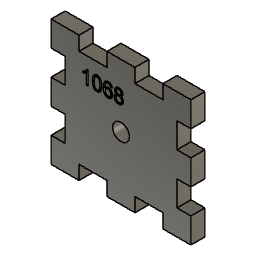
FullSystemAssembly (Autodesk Fusion 360 archive; units mm, degrees)
design "Housing_4"
Autodesk Fusion 360 part; units mm, degrees
(part 1 of 2)
sketch "Sketch1" plane through (0, 0, 0) normal (0, 1, 0) x (1, 0, 0)
  line L0 (-40.266, -48.8623) -> (-30.266, -48.8623)
  line L1 (-30.266, -48.8623) -> (-30.266, -43.8623)
  line L2 (-35.266, -39.8623) -> (-40.266, -39.8623)
  line L3 (-40.266, -39.8623) -> (-40.266, -48.8623)
  line L4 (-20.266, -48.8623) -> (-10.266, -48.8623)
  line L5 (-10.266, -48.8623) -> (-10.266, -43.8623)
  line L6 (-20.266, -43.8623) -> (-20.266, -48.8623)
  line L7 (-40.266, -30.8623) -> (-35.266, -30.8623)
  line L8 (-35.266, -21.8623) -> (-40.266, -21.8623)
  line L9 (-40.266, -21.8623) -> (-40.266, -30.8623)
  line L10 (-15.266, -66.877) -> (-15.266, -0.0799) construction
  line L11 (24.5212, -26.3623) -> (-48.7253, -26.3623) construction
  line L12 (4.734, -39.8623) -> (9.734, -39.8623)
  line L13 (-0.266, -48.8623) -> (-0.266, -43.8623)
  line L14 (9.734, -30.8623) -> (4.734, -30.8623)
  line L15 (4.734, -21.8623) -> (9.734, -21.8623)
  line L16 (-35.266, -12.8623) -> (-40.266, -12.8623)
  line L17 (-30.266, -3.8623) -> (-30.266, -8.8623)
  line L18 (-20.266, -8.8623) -> (-20.266, -3.8623)
  line L19 (-10.266, -3.8623) -> (-10.266, -8.8623)
  line L20 (-0.266, -3.8623) -> (-0.266, -8.8623)
  line L21 (4.734, -12.8623) -> (9.734, -12.8623)
  line L22 (-40.266, -48.8623) -> (-30.266, -48.8623)
  line L23 (-20.266, -48.8623) -> (-10.266, -48.8623)
  line L24 (-0.266, -48.8623) -> (9.734, -48.8623)
  line L25 (9.734, -48.8623) -> (9.734, -39.8623)
  line L26 (9.734, -30.8623) -> (9.734, -21.8623)
  line L27 (9.734, -12.8623) -> (9.734, -3.8623)
  line L28 (-40.266, -3.8623) -> (-40.266, -12.8623)
  line L29 (-40.266, -21.8623) -> (-40.266, -30.8623)
  line L30 (-40.266, -39.8623) -> (-40.266, -48.8623)
  line L31 (-35.266, -39.8623) -> (-35.266, -30.8623)
  line L32 (-35.266, -21.8623) -> (-35.266, -12.8623)
  line L33 (4.734, -39.8623) -> (4.734, -30.8623)
  line L34 (4.734, -21.8623) -> (4.734, -12.8623)
  line L35 (9.734, -3.8623) -> (-0.266, -3.8623)
  line L36 (-10.266, -3.8623) -> (-20.266, -3.8623)
  line L37 (-30.266, -3.8623) -> (-40.266, -3.8623)
  line L38 (-30.266, -8.8623) -> (-20.266, -8.8623)
  line L39 (-10.266, -8.8623) -> (-0.266, -8.8623)
  line L40 (-30.266, -43.8623) -> (-20.266, -43.8623)
  line L41 (-10.266, -43.8623) -> (-0.266, -43.8623)
  dimension "d1" = 50
  dimension "d2" = 45
  dimension "d3" = 10
  dimension "d4" = 9
  dimension "d5" = 10
  dimension "d6" = 10
  dimension "d7" = 5
  dimension "d8" = 9
  dimension "d9" = 5
  dimension "d10" = 9
  constraint horizontal L22
  constraint vertical L25
  constraint horizontal L35
  constraint vertical L28
  constraint horizontal L0
  constraint vertical L1
  constraint horizontal L2
  constraint vertical L3
  constraint horizontal L4
  constraint vertical L5
  constraint vertical L6
  constraint horizontal L7
  constraint horizontal L8
  constraint vertical L9
  constraint perpendicular L10 L35
  constraint perpendicular L11 L28
  constraint symmetric L0.end L10 L13.start
  constraint symmetric L2.end L10 L12.end
  constraint symmetric L7.start L10 L14.start
  constraint symmetric L7.end L10 L14.end
  constraint symmetric L8.start L10 L15.start
  constraint symmetric L8.end L10 L15.end
  constraint symmetric L0.end L11 L17.start
  constraint symmetric L2.end L11 L16.end
  constraint symmetric L4.start L11 L18.end
  constraint symmetric L4.end L11 L19.start
  constraint symmetric L5.end L11 L19.end
  constraint symmetric L6.start L11 L18.start
  constraint symmetric L11 L12.end L21.end
  constraint symmetric L11 L13.start L20.start
  constraint perpendicular L16 L31
  constraint perpendicular L21 L33
  constraint perpendicular L20 L38
  constraint perpendicular L13 L40
  constraint collinear L22 L23
  constraint collinear L23 L24
  constraint collinear L25 L26
  constraint collinear L26 L27
  constraint collinear L28 L29
  constraint collinear L29 L30
  constraint collinear L31 L32
  constraint collinear L33 L34
  constraint collinear L35 L36
  constraint collinear L36 L37
  constraint collinear L38 L39
  constraint collinear L40 L41
  measures "d1" distance of L0.start L24.end
  measures "d2" distance of L0.start L28.start
  measures "d3" distance of L0.start L0.end
  measures "d4" distance of L0.start L2.end
  measures "d5" distance of L0.end L4.start
  measures "d6" distance of L4.start L4.end
  measures "d7" distance of L4.start L6.start
  measures "d8" distance of L2.end L7.start
  measures "d9" distance of L7.start L7.end
  measures "d10" distance of L7.start L8.end
extrude "Extrude1" add sketch "Sketch1" along normal blind 5
sketch "Sketch2" plane through (0, 0, 0) normal (0, -1, 0) x (1, 0, 0)
  line L0 (-40.266, 39.8623) -> (-35.266, 39.8623)
  line L1 (-35.266, 39.8623) -> (-35.266, 30.8623)
  line L2 (-35.266, 30.8623) -> (-40.266, 30.8623)
  line L3 (-40.266, 30.8623) -> (-40.266, 21.8623)
  line L4 (-40.266, 21.8623) -> (-35.266, 21.8623)
  line L5 (-35.266, 21.8623) -> (-35.266, 12.8623)
  line L6 (-35.266, 12.8623) -> (-40.266, 12.8623)
  line L7 (-40.266, 12.8623) -> (-40.266, 3.8623)
  line L8 (-40.266, 3.8623) -> (-30.266, 3.8623)
  line L9 (-30.266, 3.8623) -> (-30.266, 8.8623)
  line L10 (-30.266, 8.8623) -> (-20.266, 8.8623)
  line L11 (-20.266, 8.8623) -> (-20.266, 3.8623)
  line L12 (-20.266, 3.8623) -> (-10.266, 3.8623)
  line L13 (-10.266, 3.8623) -> (-10.266, 8.8623)
  line L14 (-10.266, 8.8623) -> (-0.266, 8.8623)
  line L15 (-0.266, 8.8623) -> (-0.266, 3.8623)
  line L16 (-0.266, 3.8623) -> (9.734, 3.8623)
  line L17 (9.734, 3.8623) -> (9.734, 12.8623)
  line L18 (9.734, 12.8623) -> (4.734, 12.8623)
  line L19 (4.734, 12.8623) -> (4.734, 21.8623)
  line L20 (4.734, 21.8623) -> (9.734, 21.8623)
  line L21 (9.734, 21.8623) -> (9.734, 30.8623)
  line L22 (9.734, 30.8623) -> (4.734, 30.8623)
  line L23 (4.734, 30.8623) -> (4.734, 39.8623)
  line L24 (4.734, 39.8623) -> (9.734, 39.8623)
  line L25 (9.734, 39.8623) -> (9.734, 48.8623)
  line L26 (9.734, 48.8623) -> (-0.266, 48.8623)
  line L27 (-0.266, 48.8623) -> (-0.266, 43.8623)
  line L28 (-0.266, 43.8623) -> (-10.266, 43.8623)
  line L29 (-10.266, 43.8623) -> (-10.266, 48.8623)
  line L30 (-10.266, 48.8623) -> (-20.266, 48.8623)
  line L31 (-20.266, 48.8623) -> (-20.266, 43.8623)
  line L32 (-20.266, 43.8623) -> (-30.266, 43.8623)
  line L33 (-30.266, 43.8623) -> (-30.266, 48.8623)
  line L34 (-30.266, 48.8623) -> (-40.266, 48.8623)
  line L35 (-40.266, 48.8623) -> (-40.266, 39.8623)
  circle A0 centre (-15.266, 26.3623) radius 3
  dimension "d13" = 6
  dimension "d14" = 22.5
  dimension "d15" = 25
  measures "d13" diameter of A0
  measures "d14" distance of L12 A0.centre
  measures "d15" distance of L3 A0.centre
extrude "Extrude2" cut sketch "Sketch2" against normal blind 5 contours A0
sketch "Sketch3" plane through (0, 0, 0) normal (0, -1, 0) x (1, 0, 0)
  circle A0 centre (-15.266, 26.3623) radius 3
  line L0 (-40.266, 39.8623) -> (-35.266, 39.8623)
  line L1 (-35.266, 39.8623) -> (-35.266, 30.8623)
  line L2 (-35.266, 30.8623) -> (-40.266, 30.8623)
  line L3 (-40.266, 30.8623) -> (-40.266, 21.8623)
  line L4 (-40.266, 21.8623) -> (-35.266, 21.8623)
  line L5 (-35.266, 21.8623) -> (-35.266, 12.8623)
  line L6 (-35.266, 12.8623) -> (-40.266, 12.8623)
  line L7 (-40.266, 12.8623) -> (-40.266, 3.8623)
  line L8 (-40.266, 3.8623) -> (-30.266, 3.8623)
  line L9 (-30.266, 3.8623) -> (-30.266, 8.8623)
  line L10 (-30.266, 8.8623) -> (-20.266, 8.8623)
  line L11 (-20.266, 8.8623) -> (-20.266, 3.8623)
  line L12 (-20.266, 3.8623) -> (-10.266, 3.8623)
  line L13 (-10.266, 3.8623) -> (-10.266, 8.8623)
  line L14 (-10.266, 8.8623) -> (-0.266, 8.8623)
  line L15 (-0.266, 8.8623) -> (-0.266, 3.8623)
  line L16 (-0.266, 3.8623) -> (9.734, 3.8623)
  line L17 (9.734, 3.8623) -> (9.734, 12.8623)
  line L18 (9.734, 12.8623) -> (4.734, 12.8623)
  line L19 (4.734, 12.8623) -> (4.734, 21.8623)
  line L20 (4.734, 21.8623) -> (9.734, 21.8623)
  line L21 (9.734, 21.8623) -> (9.734, 30.8623)
  line L22 (9.734, 30.8623) -> (4.734, 30.8623)
  line L23 (4.734, 30.8623) -> (4.734, 39.8623)
  line L24 (4.734, 39.8623) -> (9.734, 39.8623)
  line L25 (9.734, 39.8623) -> (9.734, 48.8623)
  line L26 (9.734, 48.8623) -> (-0.266, 48.8623)
  line L27 (-0.266, 48.8623) -> (-0.266, 43.8623)
  line L28 (-0.266, 43.8623) -> (-10.266, 43.8623)
  line L29 (-10.266, 43.8623) -> (-10.266, 48.8623)
  line L30 (-10.266, 48.8623) -> (-20.266, 48.8623)
  line L31 (-20.266, 48.8623) -> (-20.266, 43.8623)
  line L32 (-20.266, 43.8623) -> (-30.266, 43.8623)
  line L33 (-30.266, 43.8623) -> (-30.266, 48.8623)
  line L34 (-30.266, 48.8623) -> (-40.266, 48.8623)
  line L35 (-40.266, 48.8623) -> (-40.266, 39.8623)
  line L36 (-28.8758, 34.3033) -> (-13.6356, 34.3033) construction
  line L37 (-13.6356, 34.3033) -> (-13.6356, 39.6747) construction
  line L38 (-13.6356, 39.6747) -> (-28.8758, 39.6747) construction
  line L39 (-28.8758, 39.6747) -> (-28.8758, 34.3033) construction
  dimension "d18" = 5
  text T0 "1068" font "Arial" height 5 align left top in box 15.2402 x 5.3713 at (-28.8758, 34.3033) x (1, 0) y (0, 1) spacing 1 kerned
emboss "Emboss1" depth -0.7 profiles "Sketch3" section 1 text T0 onto face at (-2.7731, 0, 18.4656)

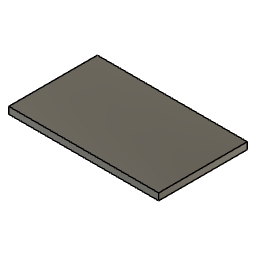
design "Base Plate"
Autodesk Fusion 360 part; units mm, degrees
sketch "Sketch1" plane through (0, 0, 0) normal (0, 0, 1) x (1, 0, 0)
  line L0 (-61.3423, 35.855) -> (48.6577, 35.855)
  line L1 (48.6577, 35.855) -> (48.6577, -29.145)
  line L2 (48.6577, -29.145) -> (-61.3423, -29.145)
  line L3 (-61.3423, -29.145) -> (-61.3423, 35.855)
  dimension "d1" = 110
  dimension "d2" = 65
  constraint horizontal L0
  constraint vertical L1
  constraint horizontal L2
  constraint vertical L3
  measures "d1" distance of L0.start L0.end
  measures "d2" distance of L0.start L2.end
extrude "Extrude1" add sketch "Sketch1" along normal blind 5

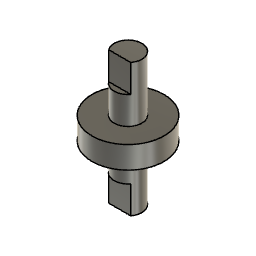
design "Shaft_bearing"
Autodesk Fusion 360 part; units mm, degrees
sketch "Sketch1" plane through (0, 0, 0) normal (0, 0, 1) x (1, 0, 0)
  circle A0 centre (0, 0) radius 6.5
  dimension "d1" = 13
  constraint coincident A0.centre origin
  measures "d1" diameter of A0
extrude "Extrude1" add sketch "Sketch1" along normal blind 4
sketch "Sketch2" plane through (0, 0, 4) normal (0, 0, 1) x (-1, 0, 0)
  circle A0 centre (0, 0) radius 6.5
  circle A1 centre (0, 0) radius 2.5
  dimension "d4" = 5
  constraint coincident A0.centre A1.centre
  measures "d4" diameter of A1
extrude "Extrude2" add sketch "Sketch2" along normal blind 5 contours A1
sketch "Sketch3" plane through (0, 0, 9) normal (0, 0, 1) x (-1, 0, 0)
  circle A0 centre (0, 0) radius 2.5
  line L0 (0, 0) -> (0, 1.5) construction
  line L1 (2, 1.5) -> (-2, 1.5)
  arc A1 (-2, 1.5) -> (2, 1.5) centre (0, 0) ccw
  dimension "d7" = 1.5
  constraint coincident A0.centre L0.start
  constraint vertical L0
  constraint perpendicular L0 L1
  constraint coincident A0 L1.start
  constraint coincident A0 L1.end
  measures "d7" distance of A0.centre L0.end
extrude "Extrude3" add sketch "Sketch3" along normal blind 5 contours A0 L1 A1
sketch "Sketch4" plane through (0, 0, 0) normal (0, 0, -1) x (1, 0, 0)
  circle A0 centre (0, 0) radius 6.5
  circle A1 centre (0, 0) radius 2.5
  dimension "d10" = 5
  constraint coincident A0.centre A1.centre
  measures "d10" diameter of A1
extrude "Extrude4" add sketch "Sketch4" along normal blind 5 contours A1
sketch "Sketch5" plane through (0, 0, -5) normal (0, 0, -1) x (1, 0, 0)
  circle A0 centre (0, 0) radius 2.5
  line L0 (0, 0) -> (0, -1.5) construction
  line L1 (2, -1.5) -> (-2, -1.5)
  arc A1 (2, -1.5) -> (-2, -1.5) centre (0, 0) ccw
  dimension "d13" = 1.5
  constraint coincident A0.centre L0.start
  constraint vertical L0
  constraint horizontal L1
  constraint coincident A0 L1.start
  constraint coincident A0 L1.end
  measures "d13" distance of A0.centre L0.end
extrude "Extrude5" add sketch "Sketch5" along normal blind 5 contours A0 L1 A1
delete_face "DeleteFace1" 1 faces at (-2.1569, 1.264, -5)
ref_plane "WorkPlane1" through (0, 0, 2) normal (0, 0, 1) x (1, 0, 0)
mirror "Mirror1" about plane through (0, 0, 2) normal (0, 0, 1) of bodies 1 merged

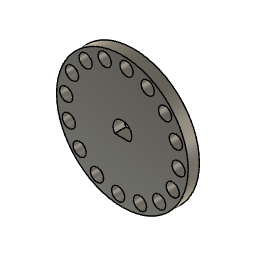
design "Slotted_disk"
Autodesk Fusion 360 part; units mm, degrees
sketch "Sketch1" plane through (0, 0, 0) normal (0, 1, 0) x (1, 0, 0)
  circle A0 centre (0, 0) radius 17.5
  line L0 (0, 0) -> (0, 1.5) construction
  line L1 (-2, 1.5) -> (2, 1.5)
  arc A1 (-2, 1.5) -> (2, 1.5) centre (0, 0) ccw
  circle A2 centre (0, 0) radius 15 construction
  circle A3 centre (-13.3942, -6.7524) radius 1.75
  circle A4 centre (-9.7906, -11.3641) radius 1.75
  circle A5 centre (-4.6965, -14.2458) radius 1.75
  circle A6 centre (1.1126, -14.9587) radius 1.75
  circle A7 centre (6.7524, -13.3942) radius 1.75
  circle A8 centre (11.3641, -9.7906) radius 1.75
  circle A9 centre (14.2458, -4.6965) radius 1.75
  circle A10 centre (14.9587, 1.1126) radius 1.75
  circle A11 centre (13.3942, 6.7524) radius 1.75
  circle A12 centre (9.7906, 11.3641) radius 1.75
  circle A13 centre (4.6965, 14.2458) radius 1.75
  circle A14 centre (-1.1126, 14.9587) radius 1.75
  circle A15 centre (-6.7524, 13.3942) radius 1.75
  circle A16 centre (-11.3641, 9.7906) radius 1.75
  circle A17 centre (-14.2458, 4.6965) radius 1.75
  circle A18 centre (-14.9587, -1.1126) radius 1.75
  dimension "d1" = 35
  dimension "d2" = 5
  dimension "d3" = 1.5
  dimension "d5" = 30
  dimension "d6" = 3.5
  dimension "d8" = 360
  constraint coincident A0.centre L0.start
  constraint concentric A0 A1
  constraint vertical L0
  constraint perpendicular L0 L1
  constraint coincident A2 A3.centre
  measures "d1" diameter of A0
  measures "d2" diameter of A1
  measures "d3" distance of A0.centre L0.end
  measures "d5" diameter of A2
  measures "d6" diameter of A3
sketch "Sketch2" plane through (0, 3, 0) normal (0, 1, 0) x (-1, 0, 0)
  circle A0 centre (10.4433, 12.1217) radius 2
  circle A1 centre (14.2872, 7.2025) radius 2
  arc A2 (2, -1.5) -> (-2, -1.5) centre (0, 0) ccw
  line L0 (2, -1.5) -> (-2, -1.5)
  circle A3 centre (-12.1217, 10.4433) radius 2
  circle A4 centre (-7.2025, 14.2872) radius 2
  circle A5 centre (-1.1868, 15.9559) radius 2
  circle A6 centre (5.0096, 15.1955) radius 2
  circle A7 centre (-15.1955, 5.0096) radius 2
  circle A8 centre (-15.9559, -1.1868) radius 2
  circle A9 centre (-14.2872, -7.2025) radius 2
  circle A10 centre (-10.4433, -12.1217) radius 2
  circle A11 centre (-5.0096, -15.1955) radius 2
  circle A12 centre (1.1868, -15.9559) radius 2
  circle A13 centre (7.2025, -14.2872) radius 2
  circle A14 centre (12.1217, -10.4433) radius 2
  circle A15 centre (15.1955, -5.0096) radius 2
  circle A16 centre (15.9559, 1.1868) radius 2
  circle A17 centre (0, 0) radius 19
  line L1 (-3.4849, 5.684) -> (8.4657, 5.2448) construction
  line L2 (8.4657, 5.2448) -> (8.6204, 9.4533) construction
  line L3 (8.6204, 9.4533) -> (-3.3303, 9.8924) construction
  line L4 (-3.3303, 9.8924) -> (-3.4849, 5.684) construction
  dimension "d11" = 4
  text T0 "1068" font "Arial" height 4 align left top in box 11.9587 x 4.2113 at (-3.4849, 5.684) x (0.999326, -0.036721) y (0.036721, 0.999326) spacing 1 kerned
extrude "Extrude2" add sketch "Sketch1" along normal blind 3
emboss "Emboss2" depth -0.5 profiles "Sketch2" section 1 text T0 onto face at (1.6994, 3, -9.1609)

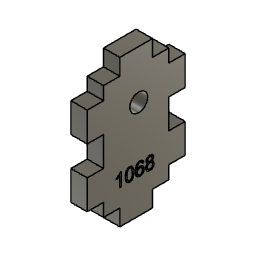
design "Housing_3"
Autodesk Fusion 360 part; units mm, degrees
sketch "Sketch1" plane through (0, 0, 0) normal (1, 0, 0) x (0, 1, 0)
  line L0 (-14.2005, 65.0328) -> (-4.2005, 65.0328)
  line L1 (-19.2005, 60.0328) -> (-19.2005, 56.0328)
  line L2 (-19.2005, 56.0328) -> (-24.2005, 56.0328)
  line L3 (-14.2005, 65.0328) -> (-14.2005, 60.0328)
  line L4 (-14.2005, 60.0328) -> (-19.2005, 60.0328)
  line L5 (-19.2005, 38.0328) -> (-24.2005, 38.0328)
  line L6 (-19.2005, 42.5328) -> (-19.2005, 38.0328)
  line L7 (-19.2005, 42.5328) -> (-19.2005, 47.0328)
  line L8 (-24.2005, 47.0328) -> (-19.2005, 47.0328)
  line L9 (-19.2005, 25.0328) -> (-19.2005, 27.5328)
  line L10 (-9.2005, 80.7683) -> (-9.2005, 14.0865) construction
  line L11 (-40.7163, 42.5328) -> (11.7648, 42.5328) construction
  line L12 (-4.2005, 60.0328) -> (0.7995, 60.0328)
  line L13 (-4.2005, 65.0328) -> (-4.2005, 60.0328)
  line L14 (0.7995, 60.0328) -> (0.7995, 56.0328)
  line L15 (0.7995, 56.0328) -> (5.7995, 56.0328)
  line L16 (5.7995, 47.0328) -> (0.7995, 47.0328)
  line L17 (0.7995, 42.5328) -> (0.7995, 47.0328)
  line L18 (0.7995, 42.5328) -> (0.7995, 38.0328)
  line L19 (0.7995, 38.0328) -> (5.7995, 38.0328)
  line L20 (-14.2005, 25.0328) -> (-19.2005, 25.0328)
  line L21 (-14.2005, 20.0328) -> (-14.2005, 25.0328)
  line L22 (-19.2005, 25.0328) -> (-19.2005, 29.0328)
  line L23 (-19.2005, 29.0328) -> (-24.2005, 29.0328)
  line L24 (-4.2005, 20.0328) -> (-4.2005, 25.0328)
  line L25 (-4.2005, 25.0328) -> (0.7995, 25.0328)
  line L26 (0.7995, 25.0328) -> (0.7995, 29.0328)
  line L27 (0.7995, 29.0328) -> (5.7995, 29.0328)
  line L28 (5.7995, 56.0328) -> (5.7995, 47.0328)
  line L29 (5.7995, 38.0328) -> (5.7995, 29.0328)
  line L30 (-4.2005, 20.0328) -> (-14.2005, 20.0328)
  line L31 (-24.2005, 29.0328) -> (-24.2005, 38.0328)
  line L32 (-24.2005, 47.0328) -> (-24.2005, 56.0328)
  line L33 (-4.2005, 65.0328) -> (-4.2005, 60.0328)
  line L34 (-4.2005, 60.0328) -> (0.7995, 60.0328)
  line L35 (0.7995, 56.0328) -> (5.7995, 56.0328)
  line L36 (0.7995, 60.0328) -> (0.7995, 56.0328)
  line L37 (5.7995, 47.0328) -> (5.7995, 56.0328)
  line L38 (5.7995, 47.0328) -> (0.7995, 47.0328)
  line L39 (0.7995, 42.5328) -> (0.7995, 47.0328)
  line L40 (-14.2005, 20.0328) -> (-14.2005, 25.0328)
  line L41 (-14.2005, 20.0328) -> (-4.2005, 20.0328)
  line L42 (-4.2005, 20.0328) -> (-4.2005, 25.0328)
  line L43 (-4.2005, 25.0328) -> (0.7995, 25.0328)
  line L44 (0.7995, 25.0328) -> (0.7995, 29.0328)
  line L45 (0.7995, 29.0328) -> (5.7995, 29.0328)
  line L46 (5.7995, 38.0328) -> (5.7995, 29.0328)
  line L47 (0.7995, 42.5328) -> (0.7995, 38.0328)
  line L48 (-19.2005, 42.5328) -> (-19.2005, 38.0328)
  line L49 (-24.2005, 38.0328) -> (-24.2005, 29.0328)
  line L50 (-19.2005, 29.0328) -> (-24.2005, 29.0328)
  line L51 (-19.2005, 25.0328) -> (-19.2005, 29.0328)
  line L52 (-14.2005, 25.0328) -> (-19.2005, 25.0328)
  dimension "d13" = 45
  dimension "d14" = 9
  dimension "d15" = 4
  dimension "d17" = 9
  dimension "d18" = 9
  constraint horizontal L0
  constraint vertical L28
  constraint horizontal L30
  constraint vertical L31
  constraint vertical L1
  constraint horizontal L2
  constraint vertical L3
  constraint horizontal L4
  constraint perpendicular L10 L30
  constraint perpendicular L11 L28
  constraint symmetric L1.end L10 L14.end
  constraint symmetric L2.end L10 L15.end
  constraint symmetric L0.start L10 L0.end
  constraint symmetric L3.end L10 L12.start
  constraint symmetric L1.start L10 L12.end
  constraint symmetric L5.start L10 L18.end
  constraint symmetric L5.end L10 L19.end
  constraint symmetric L6.start L10 L17.start
  constraint symmetric L7.end L10 L16.end
  constraint symmetric L8.start L10 L16.start
  constraint symmetric L1.end L11 L22.end
  constraint symmetric L2.end L11 L23.end
  constraint symmetric L0.start L11 L21.start
  constraint symmetric L3.end L11 L20.start
  constraint symmetric L1.start L11 L9.start
  constraint symmetric L11 L12.start L24.end
  constraint symmetric L11 L12.end L25.end
  constraint symmetric L11 L0.end L24.start
  constraint symmetric L11 L14.end L26.end
  constraint symmetric L11 L15.end L27.end
  constraint collinear L28 L29
  constraint collinear L31 L32
  constraint symmetric L6.start L11 L7.start
  constraint symmetric L7.end L11 L5.start
  constraint symmetric L11 L16.end L18.end
  constraint symmetric L11 L17.start L18.start
  measures "d13" distance of L0 L30
  measures "d14" distance of L0 L2
  measures "d15" distance of L2 L4
  measures "d17" distance of L2 L8
  measures "d18" distance of L5 L50
extrude "Extrude1" add sketch "Sketch1" along normal blind 5
sketch "Sketch2" plane through (5, 0, 0) normal (1, 0, 0) x (0, 1, 0)
  line L0 (-19.2005, 47.0328) -> (-19.2005, 38.0328)
  line L1 (-19.2005, 38.0328) -> (-24.2005, 38.0328)
  line L2 (-24.2005, 38.0328) -> (-24.2005, 29.0328)
  line L3 (-24.2005, 29.0328) -> (-19.2005, 29.0328)
  line L4 (-19.2005, 29.0328) -> (-19.2005, 25.0328)
  line L5 (-19.2005, 25.0328) -> (-14.2005, 25.0328)
  line L6 (-14.2005, 25.0328) -> (-14.2005, 20.0328)
  line L7 (-14.2005, 20.0328) -> (-4.2005, 20.0328)
  line L8 (-4.2005, 20.0328) -> (-4.2005, 25.0328)
  line L9 (-4.2005, 25.0328) -> (0.7995, 25.0328)
  line L10 (0.7995, 25.0328) -> (0.7995, 29.0328)
  line L11 (0.7995, 29.0328) -> (5.7995, 29.0328)
  line L12 (5.7995, 29.0328) -> (5.7995, 38.0328)
  line L13 (5.7995, 38.0328) -> (0.7995, 38.0328)
  line L14 (0.7995, 38.0328) -> (0.7995, 47.0328)
  line L15 (0.7995, 47.0328) -> (5.7995, 47.0328)
  line L16 (5.7995, 47.0328) -> (5.7995, 56.0328)
  line L17 (5.7995, 56.0328) -> (0.7995, 56.0328)
  line L18 (0.7995, 56.0328) -> (0.7995, 60.0328)
  line L19 (0.7995, 60.0328) -> (-4.2005, 60.0328)
  line L20 (-4.2005, 60.0328) -> (-4.2005, 65.0328)
  line L21 (-4.2005, 65.0328) -> (-14.2005, 65.0328)
  line L22 (-14.2005, 65.0328) -> (-14.2005, 60.0328)
  line L23 (-14.2005, 60.0328) -> (-19.2005, 60.0328)
  line L24 (-19.2005, 60.0328) -> (-19.2005, 56.0328)
  line L25 (-19.2005, 56.0328) -> (-24.2005, 56.0328)
  line L26 (-24.2005, 56.0328) -> (-24.2005, 47.0328)
  line L27 (-24.2005, 47.0328) -> (-19.2005, 47.0328)
  line L28 (-15.2384, 29.0856) -> (-1.443, 29.0856) construction
  line L29 (-1.443, 29.0856) -> (-1.443, 34.4691) construction
  line L30 (-1.443, 34.4691) -> (-15.2384, 34.4691) construction
  line L31 (-15.2384, 34.4691) -> (-15.2384, 29.0856) construction
  dimension "d19" = 4
  text T0 "1068" font "Arial" height 4 align left top in box 13.7954 x 5.3836 at (-15.2384, 29.0856) x (1, 0) y (0, 1) spacing 1 kerned
emboss "Emboss1" depth -0.7 profiles "Sketch2" section 1 text T0 onto face at (5, -7.5339, 51.3662)
sketch "Sketch3" plane through (5, 0, 0) normal (1, 0, 0) x (0, 1, 0)
  spline S0 degree 3 poles (-6.2971, 31.626) (-6.2904, 31.7485) (-6.2778, 31.9829) (-6.1569, 32.1837) (-6.0993, 32.2795) knots 0 0 0 0 0.036185 0.069208 0.069208 0.069208 0.069208
  spline S1 degree 3 poles (-6.0993, 32.2795) (-6.0242, 32.3608) (-5.8682, 32.5297) (-5.6494, 32.6012) (-5.5358, 32.6383) knots 0 0 0 0 0.032632 0.067797 0.067797 0.067797 0.067797
  spline S2 degree 3 poles (-5.5358, 32.6383) (-5.6292, 32.677) (-5.8045, 32.7497) (-5.9301, 32.8913) (-5.9888, 32.9575) knots 0 0 0 0 0.029866 0.056058 0.056058 0.056058 0.056058
  spline S3 degree 3 poles (-5.9888, 32.9575) (-6.0317, 33.0316) (-6.1207, 33.1851) (-6.1308, 33.3624) (-6.1361, 33.4541) knots 0 0 0 0 0.025322 0.052449 0.052449 0.052449 0.052449
  spline S4 degree 3 poles (-6.1361, 33.4541) (-6.1232, 33.5937) (-6.0974, 33.8721) (-5.9138, 34.0829) (-5.8223, 34.1881) knots 0 0 0 0 0.040936 0.081647 0.081647 0.081647 0.081647
  spline S5 degree 3 poles (-5.8223, 34.1881) (-5.705, 34.2748) (-5.4575, 34.4576) (-5.1494, 34.4759) (-4.9874, 34.4855) knots 0 0 0 0 0.042829 0.090345 0.090345 0.090345 0.090345
  spline S6 degree 3 poles (-4.9874, 34.4855) (-4.8241, 34.4754) (-4.5125, 34.4562) (-4.2631, 34.2699) (-4.1443, 34.1812) knots 0 0 0 0 0.04788 0.091383 0.091383 0.091383 0.091383
  spline S7 degree 3 poles (-4.1443, 34.1812) (-4.0512, 34.0745) (-3.8655, 33.8617) (-3.8385, 33.5806) (-3.825, 33.4405) knots 0 0 0 0 0.041365 0.082494 0.082494 0.082494 0.082494
  spline S8 degree 3 poles (-3.825, 33.4405) (-3.8305, 33.3517) (-3.841, 33.1786) (-3.9284, 33.029) (-3.971, 32.9561) knots 0 0 0 0 0.026278 0.051217 0.051217 0.051217 0.051217
  spline S9 degree 3 poles (-3.971, 32.9561) (-4.0287, 32.8904) (-4.1516, 32.7504) (-4.3233, 32.6771) (-4.4144, 32.6383) knots 0 0 0 0 0.025902 0.055176 0.055176 0.055176 0.055176
  spline S10 degree 3 poles (-4.4144, 32.6383) (-4.3005, 32.5942) (-4.0822, 32.5098) (-3.9276, 32.3346) (-3.8537, 32.2508) knots 0 0 0 0 0.03603 0.069049 0.069049 0.069049 0.069049
  spline S11 degree 3 poles (-3.8537, 32.2508) (-3.7976, 32.1555) (-3.6817, 31.9586) (-3.6683, 31.7302) (-3.6613, 31.6124) knots 0 0 0 0 0.032688 0.067537 0.067537 0.067537 0.067537
  spline S12 degree 3 poles (-3.6613, 31.6124) (-3.6761, 31.4485) (-3.7056, 31.1225) (-3.9184, 30.8738) (-4.0242, 30.7501) knots 0 0 0 0 0.048067 0.09564 0.09564 0.09564 0.09564
  spline S13 degree 3 poles (-4.0242, 30.7501) (-4.1588, 30.6483) (-4.4408, 30.4351) (-4.7944, 30.4126) (-4.9792, 30.4009) knots 0 0 0 0 0.049515 0.103702 0.103702 0.103702 0.103702
  spline S14 degree 3 poles (-4.9792, 30.4009) (-5.164, 30.4127) (-5.5179, 30.4354) (-5.7996, 30.6493) (-5.9342, 30.7515) knots 0 0 0 0 0.054192 0.103761 0.103761 0.103761 0.103761
  spline S15 degree 3 poles (-5.9342, 30.7515) (-6.04, 30.8765) (-6.254, 31.1292) (-6.2826, 31.4592) (-6.2971, 31.626) knots 0 0 0 0 0.047881 0.096785 0.096785 0.096785 0.096785
  line L0 (-14.0815, 34.4855) -> (-13.765, 34.4855)
  line L1 (-13.765, 34.4855) -> (-13.765, 30.4691)
  line L2 (-13.765, 30.4691) -> (-14.2561, 30.4691)
  line L3 (-14.2561, 30.4691) -> (-14.2561, 33.5987)
  spline S16 degree 3 poles (-14.2561, 33.5987) (-14.3231, 33.5405) (-14.4682, 33.4142) (-14.6327, 33.3142) (-14.7214, 33.2604) knots 0 0 0 0 0.026577 0.057616 0.057616 0.057616 0.057616
  spline S17 degree 3 poles (-14.7214, 33.2604) (-14.8114, 33.2088) (-14.9783, 33.1132) (-15.1563, 33.0403) (-15.2384, 33.0066) knots 0 0 0 0 0.031072 0.057651 0.057651 0.057651 0.057651
  line L4 (-15.2384, 33.0066) -> (-15.2384, 33.4814)
  spline S18 degree 3 poles (-15.2384, 33.4814) (-15.1067, 33.5482) (-14.8496, 33.6786) (-14.6268, 33.8615) (-14.5181, 33.9507) knots 0 0 0 0 0.044152 0.0862 0.0862 0.0862 0.0862
  spline S19 degree 3 poles (-14.5181, 33.9507) (-14.4253, 34.0371) (-14.2551, 34.1957) (-14.1358, 34.3949) (-14.0815, 34.4855) knots 0 0 0 0 0.03782 0.069339 0.069339 0.069339 0.069339
  spline S20 degree 3 poles (-7.986, 34.4855) (-7.8383, 34.4766) (-7.5554, 34.4595) (-7.3233, 34.298) (-7.2125, 34.2208) knots 0 0 0 0 0.043447 0.083175 0.083175 0.083175 0.083175
  spline S21 degree 3 poles (-7.2125, 34.2208) (-7.1217, 34.121) (-6.9318, 33.9123) (-6.8787, 33.6345) (-6.851, 33.4896) knots 0 0 0 0 0.039681 0.082998 0.082998 0.082998 0.082998
  line L5 (-6.851, 33.4896) -> (-7.3394, 33.4514)
  spline S22 degree 3 poles (-7.3394, 33.4514) (-7.3601, 33.5372) (-7.3968, 33.6889) (-7.4861, 33.8162) (-7.5249, 33.8716) knots 0 0 0 0 0.02619 0.046291 0.046291 0.046291 0.046291
  spline S23 degree 3 poles (-7.5249, 33.8716) (-7.5953, 33.9328) (-7.7364, 34.0557) (-7.9227, 34.073) (-8.016, 34.0817) knots 0 0 0 0 0.027254 0.054638 0.054638 0.054638 0.054638
  spline S24 degree 3 poles (-8.016, 34.0817) (-8.0914, 34.0766) (-8.2395, 34.0666) (-8.3659, 33.9889) (-8.428, 33.9507) knots 0 0 0 0 0.022275 0.043813 0.043813 0.043813 0.043813
  spline S25 degree 3 poles (-8.428, 33.9507) (-8.5023, 33.8852) (-8.6591, 33.7469) (-8.7473, 33.5569) (-8.7937, 33.4568) knots 0 0 0 0 0.029374 0.062044 0.062044 0.062044 0.062044
  spline S26 degree 3 poles (-8.7937, 33.4568) (-8.8328, 33.3265) (-8.9233, 33.0254) (-8.9294, 32.7105) (-8.9328, 32.5319) knots 0 0 0 0 0.04065 0.09392 0.09392 0.09392 0.09392
  spline S27 degree 3 poles (-8.9328, 32.5319) (-8.8718, 32.6154) (-8.7533, 32.7776) (-8.582, 32.8822) (-8.499, 32.933) knots 0 0 0 0 0.030699 0.059596 0.059596 0.059596 0.059596
  spline S28 degree 3 poles (-8.499, 32.933) (-8.4128, 32.9712) (-8.2414, 33.0471) (-8.0544, 33.0583) (-7.9615, 33.0639) knots 0 0 0 0 0.028039 0.055723 0.055723 0.055723 0.055723
  spline S29 degree 3 poles (-7.9615, 33.0639) (-7.8036, 33.0486) (-7.4862, 33.0177) (-7.2459, 32.8078) (-7.1252, 32.7024) knots 0 0 0 0 0.046354 0.09317 0.09317 0.09317 0.09317
  spline S30 degree 3 poles (-7.1252, 32.7024) (-7.0245, 32.5697) (-6.8153, 32.2938) (-6.7921, 31.9476) (-6.78, 31.7679) knots 0 0 0 0 0.04886 0.101584 0.101584 0.101584 0.101584
  spline S31 degree 3 poles (-6.78, 31.7679) (-6.7865, 31.6452) (-6.7993, 31.4022) (-6.895, 31.1786) (-6.9424, 31.068) knots 0 0 0 0 0.036549 0.072347 0.072347 0.072347 0.072347
  spline S32 degree 3 poles (-6.9424, 31.068) (-7.0004, 30.9672) (-7.1139, 30.7702) (-7.2984, 30.6376) (-7.3885, 30.5728) knots 0 0 0 0 0.034442 0.067338 0.067338 0.067338 0.067338
  spline S33 degree 3 poles (-7.3885, 30.5728) (-7.4875, 30.5227) (-7.6899, 30.4202) (-7.9166, 30.4074) (-8.0324, 30.4009) knots 0 0 0 0 0.032916 0.067292 0.067292 0.067292 0.067292
  spline S34 degree 3 poles (-8.0324, 30.4009) (-8.227, 30.419) (-8.6128, 30.455) (-8.8943, 30.7208) (-9.0338, 30.8525) knots 0 0 0 0 0.056862 0.112709 0.112709 0.112709 0.112709
  spline S35 degree 3 poles (-9.0338, 30.8525) (-9.1462, 31.0473) (-9.41, 31.5046) (-9.4171, 32.0359) (-9.4212, 32.3409) knots 0 0 0 0 0.066476 0.156053 0.156053 0.156053 0.156053
  spline S36 degree 3 poles (-9.4212, 32.3409) (-9.416, 32.6832) (-9.407, 33.2826) (-9.1172, 33.8036) (-8.9928, 34.0271) knots 0 0 0 0 0.100707 0.176355 0.176355 0.176355 0.176355
  spline S37 degree 3 poles (-8.9928, 34.0271) (-8.8554, 34.1608) (-8.5751, 34.4335) (-8.1849, 34.4679) (-7.986, 34.4855) knots 0 0 0 0 0.055729 0.113694 0.113694 0.113694 0.113694
  spline S38 degree 3 poles (-11.2029, 30.4009) (-11.3839, 30.4164) (-11.7369, 30.4465) (-11.9888, 30.6947) (-12.1115, 30.8156) knots 0 0 0 0 0.052668 0.102727 0.102727 0.102727 0.102727
  spline S39 degree 3 poles (-12.1115, 30.8156) (-12.2263, 31.0301) (-12.4964, 31.5349) (-12.5032, 32.1107) (-12.5072, 32.4418) knots 0 0 0 0 0.072018 0.169519 0.169519 0.169519 0.169519
  spline S40 degree 3 poles (-12.5072, 32.4418) (-12.5043, 32.6565) (-12.4991, 33.0431) (-12.4036, 33.4173) (-12.3612, 33.5837) knots 0 0 0 0 0.064122 0.115473 0.115473 0.115473 0.115473
  spline S41 degree 3 poles (-12.3612, 33.5837) (-12.3095, 33.7172) (-12.2115, 33.9704) (-12.0186, 34.1608) (-11.9274, 34.2508) knots 0 0 0 0 0.042382 0.080384 0.080384 0.080384 0.080384
  spline S42 degree 3 poles (-11.9274, 34.2508) (-11.8223, 34.3192) (-11.6024, 34.4623) (-11.3399, 34.4775) (-11.2029, 34.4855) knots 0 0 0 0 0.036962 0.077329 0.077329 0.077329 0.077329
  spline S43 degree 3 poles (-11.2029, 34.4855) (-11.1007, 34.481) (-10.9043, 34.4724) (-10.7244, 34.3937) (-10.6381, 34.3559) knots 0 0 0 0 0.030392 0.058395 0.058395 0.058395 0.058395
  spline S44 degree 3 poles (-10.6381, 34.3559) (-10.5603, 34.3073) (-10.4025, 34.2088) (-10.2927, 34.0584) (-10.237, 33.9821) knots 0 0 0 0 0.027238 0.055282 0.055282 0.055282 0.055282
  spline S45 degree 3 poles (-10.237, 33.9821) (-10.1864, 33.8933) (-10.0792, 33.7054) (-10.02, 33.4971) (-9.9888, 33.3873) knots 0 0 0 0 0.030541 0.064666 0.064666 0.064666 0.064666
  spline S46 degree 3 poles (-9.9888, 33.3873) (-9.9626, 33.2504) (-9.9029, 32.9383) (-9.9002, 32.6204) (-9.8987, 32.4418) knots 0 0 0 0 0.041717 0.095141 0.095141 0.095141 0.095141
  spline S47 degree 3 poles (-9.8987, 32.4418) (-9.9016, 32.2286) (-9.9069, 31.8439) (-10.0013, 31.4714) (-10.0433, 31.3054) knots 0 0 0 0 0.063711 0.114907 0.114907 0.114907 0.114907
  spline S48 degree 3 poles (-10.0433, 31.3054) (-10.0947, 31.1718) (-10.1921, 30.9183) (-10.3847, 30.7273) (-10.4758, 30.6369) knots 0 0 0 0 0.042369 0.080425 0.080425 0.080425 0.080425
  spline S49 degree 3 poles (-10.4758, 30.6369) (-10.5811, 30.5681) (-10.8017, 30.424) (-11.0652, 30.4088) (-11.2029, 30.4009) knots 0 0 0 0 0.037071 0.077645 0.077645 0.077645 0.077645
  line L6 (-19.2005, 47.0328) -> (-19.2005, 38.0328)
  line L7 (-19.2005, 38.0328) -> (-24.2005, 38.0328)
  line L8 (-24.2005, 38.0328) -> (-24.2005, 29.0328)
  line L9 (-24.2005, 29.0328) -> (-19.2005, 29.0328)
  line L10 (-19.2005, 29.0328) -> (-19.2005, 25.0328)
  line L11 (-19.2005, 25.0328) -> (-14.2005, 25.0328)
  line L12 (-14.2005, 25.0328) -> (-14.2005, 20.0328)
  line L13 (-14.2005, 20.0328) -> (-4.2005, 20.0328)
  line L14 (-4.2005, 20.0328) -> (-4.2005, 25.0328)
  line L15 (-4.2005, 25.0328) -> (0.7995, 25.0328)
  line L16 (0.7995, 25.0328) -> (0.7995, 29.0328)
  line L17 (0.7995, 29.0328) -> (5.7995, 29.0328)
  line L18 (5.7995, 29.0328) -> (5.7995, 38.0328)
  line L19 (5.7995, 38.0328) -> (0.7995, 38.0328)
  line L20 (0.7995, 38.0328) -> (0.7995, 47.0328)
  line L21 (0.7995, 47.0328) -> (5.7995, 47.0328)
  line L22 (5.7995, 47.0328) -> (5.7995, 56.0328)
  line L23 (5.7995, 56.0328) -> (0.7995, 56.0328)
  line L24 (0.7995, 56.0328) -> (0.7995, 60.0328)
  line L25 (0.7995, 60.0328) -> (-4.2005, 60.0328)
  line L26 (-4.2005, 60.0328) -> (-4.2005, 65.0328)
  line L27 (-4.2005, 65.0328) -> (-14.2005, 65.0328)
  line L28 (-14.2005, 65.0328) -> (-14.2005, 60.0328)
  line L29 (-14.2005, 60.0328) -> (-19.2005, 60.0328)
  line L30 (-19.2005, 60.0328) -> (-19.2005, 56.0328)
  line L31 (-19.2005, 56.0328) -> (-24.2005, 56.0328)
  line L32 (-24.2005, 56.0328) -> (-24.2005, 47.0328)
  line L33 (-24.2005, 47.0328) -> (-19.2005, 47.0328)
  circle A0 centre (-8.399, 50.2042) radius 2.75
  dimension "d24" = 5.5
  measures "d24" diameter of A0
extrude "Extrude2" cut sketch "Sketch3" against normal blind 5 contours A0

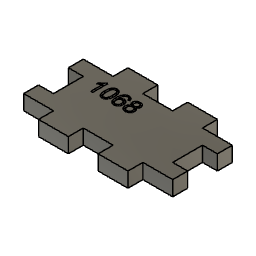
design "Housing_2"
Autodesk Fusion 360 part; units mm, degrees
sketch "Sketch1" plane through (0, 0, 0) normal (0, 0, 1) x (1, 0, 0)
  line L0 (-42.9407, 21.9767) -> (-42.9407, 26.9767)
  line L1 (-42.9407, 26.9767) -> (-52.9407, 26.9767)
  line L2 (-52.9407, 26.9767) -> (-52.9407, 31.9767)
  line L3 (-52.9407, 31.9767) -> (-47.9407, 31.9767)
  line L4 (-47.9407, 31.9767) -> (-47.9407, 41.9767)
  line L5 (-47.9407, 41.9767) -> (-52.9407, 41.9767)
  line L6 (-32.9407, 26.9767) -> (-32.9407, 21.9767)
  line L7 (-22.9407, 26.9767) -> (-32.9407, 26.9767)
  line L8 (-22.9407, 21.9767) -> (-22.9407, 26.9767)
  line L9 (-12.9407, 26.9767) -> (-12.9407, 21.9767)
  line L10 (-2.9407, 26.9767) -> (-12.9407, 26.9767)
  line L11 (-27.9407, 12.4409) -> (-27.9407, 59.643) construction
  line L12 (-59.1616, 36.9767) -> (4.5103, 36.9767) construction
  line L13 (-42.9407, 46.9767) -> (-52.9407, 46.9767)
  line L14 (-42.9407, 51.9767) -> (-42.9407, 46.9767)
  line L15 (-32.9407, 46.9767) -> (-32.9407, 51.9767)
  line L16 (-22.9407, 46.9767) -> (-32.9407, 46.9767)
  line L17 (-22.9407, 51.9767) -> (-22.9407, 46.9767)
  line L18 (-12.9407, 46.9767) -> (-12.9407, 51.9767)
  line L19 (-2.9407, 46.9767) -> (-12.9407, 46.9767)
  line L20 (-7.9407, 31.9767) -> (-7.9407, 41.9767)
  line L21 (-7.9407, 41.9767) -> (-2.9407, 41.9767)
  line L22 (-2.9407, 31.9767) -> (-7.9407, 31.9767)
  line L23 (-42.9407, 51.9767) -> (-32.9407, 51.9767)
  line L24 (-22.9407, 51.9767) -> (-12.9407, 51.9767)
  line L25 (-52.9407, 26.9767) -> (-52.9407, 31.9767)
  line L26 (-52.9407, 41.9767) -> (-52.9407, 46.9767)
  line L27 (-12.9407, 21.9767) -> (-22.9407, 21.9767)
  line L28 (-32.9407, 21.9767) -> (-42.9407, 21.9767)
  line L29 (-2.9407, 46.9767) -> (-2.9407, 41.9767)
  line L30 (-2.9407, 31.9767) -> (-2.9407, 26.9767)
  dimension "d5" = 5
  dimension "d6" = 5
  dimension "d7" = 10
  dimension "d12" = 15
  dimension "d13" = 25
  constraint horizontal L23
  constraint vertical L29
  constraint horizontal L27
  constraint vertical L25
  constraint vertical L0
  constraint horizontal L1
  constraint perpendicular L1 L2
  constraint horizontal L3
  constraint vertical L4
  constraint horizontal L5
  constraint perpendicular L11 L23
  constraint perpendicular L12 L29
  constraint symmetric L0.start L12 L14.start
  constraint symmetric L0.end L12 L13.start
  constraint symmetric L1.end L12 L13.end
  constraint symmetric L6.start L12 L15.start
  constraint symmetric L6.end L12 L15.end
  constraint symmetric L7.start L12 L16.start
  constraint symmetric L8.start L12 L17.start
  constraint symmetric L9.start L12 L18.start
  constraint symmetric L9.end L12 L18.end
  constraint symmetric L10.start L12 L19.start
  constraint symmetric L2.end L11 L22.start
  constraint symmetric L3.end L11 L20.start
  constraint symmetric L4.end L11 L20.end
  constraint symmetric L5.end L11 L21.end
  constraint collinear L23 L24
  constraint collinear L25 L26
  constraint collinear L27 L28
  constraint collinear L29 L30
  measures "d5" distance of L1.end L2.end
  measures "d6" distance of L2.end L3.end
  measures "d7" distance of L2.end L5.end
  measures "d12" distance of L12 L23
  measures "d13" distance of L11 L29
extrude "Extrude1" add sketch "Sketch1" along normal blind 5
sketch "Sketch2" plane through (0, 0, 5) normal (0, 0, 1) x (-1, 0, 0)
  line L0 (7.9407, -31.9767) -> (7.9407, -41.9767)
  line L1 (7.9407, -41.9767) -> (2.9407, -41.9767)
  line L2 (2.9407, -41.9767) -> (2.9407, -46.9767)
  line L3 (2.9407, -46.9767) -> (12.9407, -46.9767)
  line L4 (12.9407, -46.9767) -> (12.9407, -51.9767)
  line L5 (12.9407, -51.9767) -> (22.9407, -51.9767)
  line L6 (22.9407, -51.9767) -> (22.9407, -46.9767)
  line L7 (22.9407, -46.9767) -> (32.9407, -46.9767)
  line L8 (32.9407, -46.9767) -> (32.9407, -51.9767)
  line L9 (32.9407, -51.9767) -> (42.9407, -51.9767)
  line L10 (42.9407, -51.9767) -> (42.9407, -46.9767)
  line L11 (42.9407, -46.9767) -> (52.9407, -46.9767)
  line L12 (52.9407, -46.9767) -> (52.9407, -41.9767)
  line L13 (52.9407, -41.9767) -> (47.9407, -41.9767)
  line L14 (47.9407, -41.9767) -> (47.9407, -31.9767)
  line L15 (47.9407, -31.9767) -> (52.9407, -31.9767)
  line L16 (52.9407, -31.9767) -> (52.9407, -26.9767)
  line L17 (52.9407, -26.9767) -> (42.9407, -26.9767)
  line L18 (42.9407, -26.9767) -> (42.9407, -21.9767)
  line L19 (42.9407, -21.9767) -> (32.9407, -21.9767)
  line L20 (32.9407, -21.9767) -> (32.9407, -26.9767)
  line L21 (32.9407, -26.9767) -> (22.9407, -26.9767)
  line L22 (22.9407, -26.9767) -> (22.9407, -21.9767)
  line L23 (22.9407, -21.9767) -> (12.9407, -21.9767)
  line L24 (12.9407, -21.9767) -> (12.9407, -26.9767)
  line L25 (12.9407, -26.9767) -> (2.9407, -26.9767)
  line L26 (2.9407, -26.9767) -> (2.9407, -31.9767)
  line L27 (2.9407, -31.9767) -> (7.9407, -31.9767)
  line L28 (43.5617, -39.2983) -> (32.0803, -39.2983) construction
  line L29 (32.0803, -39.2983) -> (32.0803, -43.9251) construction
  line L30 (32.0803, -43.9251) -> (43.5617, -43.9251) construction
  line L31 (43.5617, -43.9251) -> (43.5617, -39.2983) construction
  dimension "d16" = 5
  text T0 "1068" font "Arial" height 5 align left top in box 11.4814 x 4.6268 at (43.5617, -39.2983) x (-1, 0) y (0, -1) spacing 1 kerned
emboss "Emboss1" depth -0.7 profiles "Sketch2" section 1 text T0 onto face at (-39.6074, 33.6433, 5)

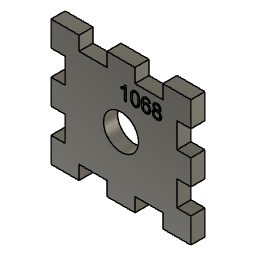
design "Housing_1"
Autodesk Fusion 360 part; units mm, degrees
sketch "Sketch1" plane through (0, 0, 0) normal (0, 1, 0) x (1, 0, 0)
  line L0 (-40.266, -48.8623) -> (-30.266, -48.8623)
  line L1 (-30.266, -48.8623) -> (-30.266, -43.8623)
  line L2 (-35.266, -39.8623) -> (-40.266, -39.8623)
  line L3 (-40.266, -39.8623) -> (-40.266, -48.8623)
  line L4 (-20.266, -48.8623) -> (-10.266, -48.8623)
  line L5 (-10.266, -48.8623) -> (-10.266, -43.8623)
  line L6 (-20.266, -43.8623) -> (-20.266, -48.8623)
  line L7 (-40.266, -30.8623) -> (-35.266, -30.8623)
  line L8 (-35.266, -21.8623) -> (-40.266, -21.8623)
  line L9 (-40.266, -21.8623) -> (-40.266, -30.8623)
  line L10 (-15.266, -66.877) -> (-15.266, -0.0799) construction
  line L11 (24.5212, -26.3623) -> (-48.7253, -26.3623) construction
  line L12 (4.734, -39.8623) -> (9.734, -39.8623)
  line L13 (-0.266, -48.8623) -> (-0.266, -43.8623)
  line L14 (9.734, -30.8623) -> (4.734, -30.8623)
  line L15 (4.734, -21.8623) -> (9.734, -21.8623)
  line L16 (-35.266, -12.8623) -> (-40.266, -12.8623)
  line L17 (-30.266, -3.8623) -> (-30.266, -8.8623)
  line L18 (-20.266, -8.8623) -> (-20.266, -3.8623)
  line L19 (-10.266, -3.8623) -> (-10.266, -8.8623)
  line L20 (-0.266, -3.8623) -> (-0.266, -8.8623)
  line L21 (4.734, -12.8623) -> (9.734, -12.8623)
  line L22 (-40.266, -48.8623) -> (-30.266, -48.8623)
  line L23 (-20.266, -48.8623) -> (-10.266, -48.8623)
  line L24 (-0.266, -48.8623) -> (9.734, -48.8623)
  line L25 (9.734, -48.8623) -> (9.734, -39.8623)
  line L26 (9.734, -30.8623) -> (9.734, -21.8623)
  line L27 (9.734, -12.8623) -> (9.734, -3.8623)
  line L28 (-40.266, -3.8623) -> (-40.266, -12.8623)
  line L29 (-40.266, -21.8623) -> (-40.266, -30.8623)
  line L30 (-40.266, -39.8623) -> (-40.266, -48.8623)
  line L31 (-35.266, -39.8623) -> (-35.266, -30.8623)
  line L32 (-35.266, -21.8623) -> (-35.266, -12.8623)
  line L33 (4.734, -39.8623) -> (4.734, -30.8623)
  line L34 (4.734, -21.8623) -> (4.734, -12.8623)
  line L35 (9.734, -3.8623) -> (-0.266, -3.8623)
  line L36 (-10.266, -3.8623) -> (-20.266, -3.8623)
  line L37 (-30.266, -3.8623) -> (-40.266, -3.8623)
  line L38 (-30.266, -8.8623) -> (-20.266, -8.8623)
  line L39 (-10.266, -8.8623) -> (-0.266, -8.8623)
  line L40 (-30.266, -43.8623) -> (-20.266, -43.8623)
  line L41 (-10.266, -43.8623) -> (-0.266, -43.8623)
  dimension "d1" = 50
  dimension "d2" = 45
  dimension "d3" = 10
  dimension "d4" = 9
  dimension "d5" = 10
  dimension "d6" = 10
  dimension "d7" = 5
  dimension "d8" = 9
  dimension "d9" = 5
  dimension "d10" = 9
  constraint horizontal L22
  constraint vertical L25
  constraint horizontal L35
  constraint vertical L28
  constraint horizontal L0
  constraint vertical L1
  constraint horizontal L2
  constraint vertical L3
  constraint horizontal L4
  constraint vertical L5
  constraint vertical L6
  constraint horizontal L7
  constraint horizontal L8
  constraint vertical L9
  constraint perpendicular L10 L35
  constraint perpendicular L11 L28
  constraint symmetric L0.end L10 L13.start
  constraint symmetric L2.end L10 L12.end
  constraint symmetric L7.start L10 L14.start
  constraint symmetric L7.end L10 L14.end
  constraint symmetric L8.start L10 L15.start
  constraint symmetric L8.end L10 L15.end
  constraint symmetric L0.end L11 L17.start
  constraint symmetric L2.end L11 L16.end
  constraint symmetric L4.start L11 L18.end
  constraint symmetric L4.end L11 L19.start
  constraint symmetric L5.end L11 L19.end
  constraint symmetric L6.start L11 L18.start
  constraint symmetric L11 L12.end L21.end
  constraint symmetric L11 L13.start L20.start
  constraint perpendicular L16 L31
  constraint perpendicular L21 L33
  constraint perpendicular L20 L38
  constraint perpendicular L13 L40
  constraint collinear L22 L23
  constraint collinear L23 L24
  constraint collinear L25 L26
  constraint collinear L26 L27
  constraint collinear L28 L29
  constraint collinear L29 L30
  constraint collinear L31 L32
  constraint collinear L33 L34
  constraint collinear L35 L36
  constraint collinear L36 L37
  constraint collinear L38 L39
  constraint collinear L40 L41
  measures "d1" distance of L0.start L24.end
  measures "d2" distance of L0.start L28.start
  measures "d3" distance of L0.start L0.end
  measures "d4" distance of L0.start L2.end
  measures "d5" distance of L0.end L4.start
  measures "d6" distance of L4.start L4.end
  measures "d7" distance of L4.start L6.start
  measures "d8" distance of L2.end L7.start
  measures "d9" distance of L7.start L7.end
  measures "d10" distance of L7.start L8.end
extrude "Extrude1" add sketch "Sketch1" along normal blind 5
sketch "Sketch2" plane through (0, 0, 0) normal (0, -1, 0) x (1, 0, 0)
  line L0 (-40.266, 39.8623) -> (-35.266, 39.8623)
  line L1 (-35.266, 39.8623) -> (-35.266, 30.8623)
  line L2 (-35.266, 30.8623) -> (-40.266, 30.8623)
  line L3 (-40.266, 30.8623) -> (-40.266, 21.8623)
  line L4 (-40.266, 21.8623) -> (-35.266, 21.8623)
  line L5 (-35.266, 21.8623) -> (-35.266, 12.8623)
  line L6 (-35.266, 12.8623) -> (-40.266, 12.8623)
  line L7 (-40.266, 12.8623) -> (-40.266, 3.8623)
  line L8 (-40.266, 3.8623) -> (-30.266, 3.8623)
  line L9 (-30.266, 3.8623) -> (-30.266, 8.8623)
  line L10 (-30.266, 8.8623) -> (-20.266, 8.8623)
  line L11 (-20.266, 8.8623) -> (-20.266, 3.8623)
  line L12 (-20.266, 3.8623) -> (-10.266, 3.8623)
  line L13 (-10.266, 3.8623) -> (-10.266, 8.8623)
  line L14 (-10.266, 8.8623) -> (-0.266, 8.8623)
  line L15 (-0.266, 8.8623) -> (-0.266, 3.8623)
  line L16 (-0.266, 3.8623) -> (9.734, 3.8623)
  line L17 (9.734, 3.8623) -> (9.734, 12.8623)
  line L18 (9.734, 12.8623) -> (4.734, 12.8623)
  line L19 (4.734, 12.8623) -> (4.734, 21.8623)
  line L20 (4.734, 21.8623) -> (9.734, 21.8623)
  line L21 (9.734, 21.8623) -> (9.734, 30.8623)
  line L22 (9.734, 30.8623) -> (4.734, 30.8623)
  line L23 (4.734, 30.8623) -> (4.734, 39.8623)
  line L24 (4.734, 39.8623) -> (9.734, 39.8623)
  line L25 (9.734, 39.8623) -> (9.734, 48.8623)
  line L26 (9.734, 48.8623) -> (-0.266, 48.8623)
  line L27 (-0.266, 48.8623) -> (-0.266, 43.8623)
  line L28 (-0.266, 43.8623) -> (-10.266, 43.8623)
  line L29 (-10.266, 43.8623) -> (-10.266, 48.8623)
  line L30 (-10.266, 48.8623) -> (-20.266, 48.8623)
  line L31 (-20.266, 48.8623) -> (-20.266, 43.8623)
  line L32 (-20.266, 43.8623) -> (-30.266, 43.8623)
  line L33 (-30.266, 43.8623) -> (-30.266, 48.8623)
  line L34 (-30.266, 48.8623) -> (-40.266, 48.8623)
  line L35 (-40.266, 48.8623) -> (-40.266, 39.8623)
  circle A0 centre (-15.266, 26.3623) radius 6.25
  dimension "d13" = 12.5
  dimension "d14" = 22.5
  dimension "d15" = 25
  measures "d13" diameter of A0
  measures "d14" distance of L12 A0.centre
  measures "d15" distance of L3 A0.centre
extrude "Extrude2" cut sketch "Sketch2" against normal blind 5 contours A0
sketch "Sketch3" plane through (0, 0, 0) normal (0, -1, 0) x (1, 0, 0)
  circle A0 centre (-15.266, 26.3623) radius 6.25
  line L0 (-40.266, 39.8623) -> (-35.266, 39.8623)
  line L1 (-35.266, 39.8623) -> (-35.266, 30.8623)
  line L2 (-35.266, 30.8623) -> (-40.266, 30.8623)
  line L3 (-40.266, 30.8623) -> (-40.266, 21.8623)
  line L4 (-40.266, 21.8623) -> (-35.266, 21.8623)
  line L5 (-35.266, 21.8623) -> (-35.266, 12.8623)
  line L6 (-35.266, 12.8623) -> (-40.266, 12.8623)
  line L7 (-40.266, 12.8623) -> (-40.266, 3.8623)
  line L8 (-40.266, 3.8623) -> (-30.266, 3.8623)
  line L9 (-30.266, 3.8623) -> (-30.266, 8.8623)
  line L10 (-30.266, 8.8623) -> (-20.266, 8.8623)
  line L11 (-20.266, 8.8623) -> (-20.266, 3.8623)
  line L12 (-20.266, 3.8623) -> (-10.266, 3.8623)
  line L13 (-10.266, 3.8623) -> (-10.266, 8.8623)
  line L14 (-10.266, 8.8623) -> (-0.266, 8.8623)
  line L15 (-0.266, 8.8623) -> (-0.266, 3.8623)
  line L16 (-0.266, 3.8623) -> (9.734, 3.8623)
  line L17 (9.734, 3.8623) -> (9.734, 12.8623)
  line L18 (9.734, 12.8623) -> (4.734, 12.8623)
  line L19 (4.734, 12.8623) -> (4.734, 21.8623)
  line L20 (4.734, 21.8623) -> (9.734, 21.8623)
  line L21 (9.734, 21.8623) -> (9.734, 30.8623)
  line L22 (9.734, 30.8623) -> (4.734, 30.8623)
  line L23 (4.734, 30.8623) -> (4.734, 39.8623)
  line L24 (4.734, 39.8623) -> (9.734, 39.8623)
  line L25 (9.734, 39.8623) -> (9.734, 48.8623)
  line L26 (9.734, 48.8623) -> (-0.266, 48.8623)
  line L27 (-0.266, 48.8623) -> (-0.266, 43.8623)
  line L28 (-0.266, 43.8623) -> (-10.266, 43.8623)
  line L29 (-10.266, 43.8623) -> (-10.266, 48.8623)
  line L30 (-10.266, 48.8623) -> (-20.266, 48.8623)
  line L31 (-20.266, 48.8623) -> (-20.266, 43.8623)
  line L32 (-20.266, 43.8623) -> (-30.266, 43.8623)
  line L33 (-30.266, 43.8623) -> (-30.266, 48.8623)
  line L34 (-30.266, 48.8623) -> (-40.266, 48.8623)
  line L35 (-40.266, 48.8623) -> (-40.266, 39.8623)
  line L36 (-15.2509, 35.5236) -> (-3.1076, 35.5453) construction
  line L37 (-3.1076, 35.5453) -> (-3.1185, 41.6389) construction
  line L38 (-3.1185, 41.6389) -> (-15.2618, 41.6172) construction
  line L39 (-15.2618, 41.6172) -> (-15.2509, 35.5236) construction
  dimension "d18" = 5
  text T0 "1068" font "Arial" height 5 align left top in box 12.1433 x 6.0936 at (-15.2509, 35.5236) x (0.999998, 0.001785) y (-0.001785, 0.999998) spacing 1 kerned
emboss "Emboss1" depth -0.7 profiles "Sketch3" section 1 text T0 onto face at (-28.654, 0, 17.8554)

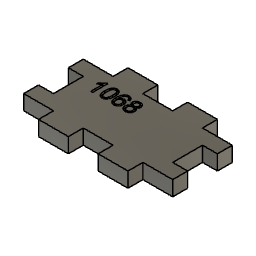
design "Housing_5"
Autodesk Fusion 360 part; units mm, degrees